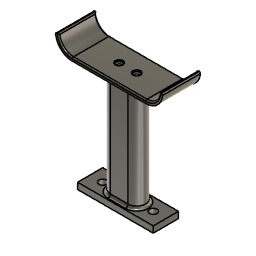
Pos7-8-9 Soporte brazal 2 (Autodesk Fusion 360 design; units mm, degrees)
Autodesk Fusion 360 part; units mm, degrees
sketch "Boceto1" plane through (0, 0, 0) normal (0, 0, 1) x (1, 0, 0)
  line L0 (-30, 10) -> (30, 10)
  line L1 (30, 10) -> (30, -10)
  line L2 (30, -10) -> (-30, -10)
  line L3 (-30, -10) -> (-30, 10)
  point P0 (0, 10)
  point P1 (-30, 0)
  dimension "d1" = 60
  dimension "d2" = 20
  constraint horizontal L0
  constraint vertical L1
  constraint horizontal L2
  constraint vertical L3
  constraint midpoint L0 P0
  constraint midpoint L3 P1
  constraint horizontal origin P1
  constraint vertical origin P0
  measures "d1" distance of L0.start L0.end
  measures "d2" distance of L0.end L1.end
extrude "Extruir1" add sketch "Boceto1" along normal blind 5 makes body 1
sketch "Boceto2" plane through (0, 0, 5) normal (0, 0, 1) x (-1, 0, 0)
  line L0 (30, 10) -> (-30, 10)
  line L1 (-30, 10) -> (-30, -10)
  line L2 (-30, -10) -> (30, -10)
  line L3 (30, -10) -> (30, 10)
  line L4 (7, 7) -> (-7, 7)
  arc A0 (-7, 7) -> (-7, -7) centre (-7, 0) ccw
  line L5 (-7, -7) -> (7, -7)
  arc A1 (7, -7) -> (7, 7) centre (7, 0) ccw
  line L6 (7, 0) -> (-7, 0) construction
  dimension "d30" = 14
  dimension "d31" = 7
  constraint tangent L4 A0
  constraint tangent A0 L5
  constraint parallel L4 L5
  constraint tangent L5 A1
  constraint tangent L4 A1
  constraint perpendicular L3 L6
  constraint midpoint L6 origin
  measures "d30" distance of A1.centre A0.centre
  measures "d31" radius of A0
extrude "Extruir2" add sketch "Boceto2" along normal blind 86 contours L4 A0 L5 A1 bodies 1
sketch "Boceto3" plane through (0, 0, 0) normal (0, 1, 0) x (1, 0, 0)
  arc A0 (42.5, -104.4096) -> (29.1237, -91.0333) centre (29.1237, -104.4096) ccw
  line L0 (29.1237, -91.0333) -> (-29.1237, -91.0333)
  arc A1 (-29.1237, -91.0333) -> (-42.5, -104.4096) centre (-29.1237, -104.4096) ccw
  line L1 (-29.1237, -104.4096) -> (29.1237, -104.4096) construction
  arc A2 (40, -104.4096) -> (29.1237, -93.5333) centre (29.1237, -104.4096) ccw
  line L2 (29.1237, -93.5333) -> (-29.1237, -93.5333)
  arc A3 (-29.1237, -93.5333) -> (-40, -104.4096) centre (-29.1237, -104.4096) ccw
  line L3 (-29.1237, -104.4096) -> (29.1237, -104.4096) construction
  line L4 (-40, -104.4096) -> (-42.5, -104.4096)
  line L5 (40, -104.4096) -> (42.5, -104.4096)
  point P0 (0, -104.4096)
  dimension "d9" = 85
  constraint tangent A0 L0
  constraint tangent L0 A1
  constraint horizontal L1
  constraint tangent A2 L2
  constraint tangent L2 A3
  constraint coincident A0.centre L1.end
  constraint parallel L1 L3
  constraint coincident A1.centre L1.start
  constraint midpoint L1 P0
  constraint vertical origin P0
  measures "d9" distance of A1.end A0.start
extrude "Extruir3" add sketch "Boceto3" along normal blind 15 and the other way blind 15 separate body makes body 2
fillet "Empalme1" radius 2 4 edges at (14, 0, 5) (0, -7, 5) (-14, 0, 5) (0, 7, 5) on bodies 1
sketch "Boceto4" plane through (0, 0, 5) normal (0, 0, 1) x (-1, 0, 0)
  line L0 (30, 10) -> (-30, 10)
  line L1 (-30, 10) -> (-30, -10)
  line L2 (-30, -10) -> (30, -10)
  line L3 (30, -10) -> (30, 10)
  circle A0 centre (20, 0) radius 3
  circle A1 centre (-20, 0) radius 3
  arc A2 (-7, 9) -> (-7, -9) centre (-7, 0) ccw
  line L4 (-7, 9) -> (7, 9)
  arc A3 (7, -9) -> (7, 9) centre (7, 0) ccw
  line L5 (7, -9) -> (-7, -9)
  dimension "d16" = 6
  dimension "d17" = 6
  dimension "d18" = 40
  constraint horizontal origin A0.centre
  constraint horizontal origin A1.centre
  measures "d16" diameter of A0
  measures "d17" diameter of A1
  measures "d18" distance of A0.centre A1.centre
extrude "Extruir4" cut sketch "Boceto4" against normal blind 10 contours A0 | A1 bodies 1
hole "Agujero1" at (7, 0, 91) direction (0, 0, -1) diameter 5.035 depth 10 tip angle 118 bodies 1
thread "Rosca1" "ISO Metric profile 6.0 M6x1 6H" thread offset 0 thread depth 7.4
hole "Agujero2" at (-7, 0, 91) direction (0, 0, -1) diameter 5.035 depth 10 tip angle 118 bodies 1
thread "Rosca2" "ISO Metric profile 6.0 M6x1 6H" thread offset 0 thread depth 7.4
fillet "Empalme2" radius 1 8 edges at (-40, 0, 104.4096) (36.8144, -15, 96.7189) (0, -15, 93.5333) (-36.8144, -15, 96.7189) (-36.8144, 15, 96.7189) (0, 15, 93.5333) (36.8144, 15, 96.7189) (40, 0, 104.4096) on bodies 2
fillet "Empalme3" radius 1 2 edges at (-42.5, 0, 104.4096) (42.5, 0, 104.4096) on bodies 2
hole "Agujero3" at (-7, 0, 93.5333) direction (0, 0, -1) diameter 5.035 depth 10 tip angle 118 counterbore diameter 6 counterbore depth 1 bodies 2
thread "Rosca3" "ISO Metric profile 6.0 M6x1 6H" thread offset 0 thread depth 7.4
mirror "Simetría1" about plane through (0, 0, 0) normal (1, 0, 0) of "Agujero3"
